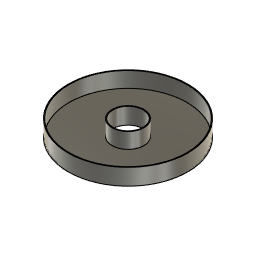
Track v2 (Autodesk Fusion 360 design; units mm, degrees)
Autodesk Fusion 360 part; units mm, degrees
note: some values were not read from the file. Set by a fixed rule: which sketch regions a step uses.
sketch "Sketch1" plane through (0, 0, 0) normal (0, 1, 0) x (1, 0, 0)
  line L0 (37, -40) -> (37, 0)
  line L1 (39, -2) -> (39, -40)
  line L2 (39, -40) -> (37, -40)
  line L3 (37, 0) -> (146.6, 0)
  line L4 (146.6, 0) -> (146.6, -40)
  line L5 (146.6, -40) -> (144.6, -40)
  line L6 (144.6, -40) -> (144.6, -2)
  line L7 (39, -2) -> (144.6, -2)
  dimension "d14" = 109.6
  dimension "d15" = 40
  dimension "d16" = 2
  dimension "d17" = 38
  constraint perpendicular L0 L3
  constraint perpendicular L3 L4
  constraint perpendicular L4 L5
  constraint perpendicular L5 L6
  constraint perpendicular L6 L7
  measures "d14" distance of L0.end L3.end
  measures "d15" distance of L3.end L4.end
  measures "d16" distance of L4.end L5.end
  measures "d17" distance of L5.end L6.end
revolve "Revolve1" add sketch "Sketch1" angle 360 about axis through (0, 0, 1.75) along (0, 0, 1)
